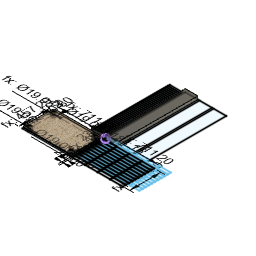
model (Autodesk Fusion 360 design; units mm, degrees)
Autodesk Fusion 360 part; units mm, degrees
sketch "Sketch1" plane through (0, 0, 0) normal (0, 0, 1) x (1, 0, 0) in component "stock"
  line L0 (0, 0) -> (184.15, 0)
  line L1 (184.15, 0) -> (184.15, 1168.4)
  line L2 (184.15, 1168.4) -> (0, 1168.4)
  line L3 (0, 1168.4) -> (0, 0)
  line L4 (-207.15, 0) -> (-23, 0)
  line L5 (-23, 0) -> (-23, 25.4)
  line L6 (-23, 25.4) -> (-207.15, 25.4)
  line L7 (-207.15, 25.4) -> (-207.15, 0)
  line L8 (-207.15, 27.4) -> (-23, 27.4)
  line L9 (-23, 27.4) -> (-23, 52.8)
  line L10 (-207.15, 52.8) -> (-207.15, 27.4)
  line L11 (-23, 52.8) -> (-207.15, 52.8)
  line L12 (-207.15, 54.8) -> (-23, 54.8)
  line L13 (-23, 54.8) -> (-23, 80.2)
  line L14 (-207.15, 80.2) -> (-207.15, 54.8)
  line L15 (-23, 80.2) -> (-207.15, 80.2)
  line L16 (-207.15, 82.2) -> (-23, 82.2)
  line L17 (-23, 82.2) -> (-23, 107.6)
  line L18 (-207.15, 107.6) -> (-207.15, 82.2)
  line L19 (-23, 107.6) -> (-207.15, 107.6)
  line L20 (-207.15, 109.6) -> (-23, 109.6)
  line L21 (-23, 109.6) -> (-23, 135)
  line L22 (-207.15, 135) -> (-207.15, 109.6)
  line L23 (-23, 135) -> (-207.15, 135)
  line L24 (-207.15, 137) -> (-23, 137)
  line L25 (-23, 137) -> (-23, 162.4)
  line L26 (-207.15, 162.4) -> (-207.15, 137)
  line L27 (-23, 162.4) -> (-207.15, 162.4)
  line L28 (-207.15, 164.4) -> (-23, 164.4)
  line L29 (-23, 164.4) -> (-23, 189.8)
  line L30 (-207.15, 189.8) -> (-207.15, 164.4)
  line L31 (-23, 189.8) -> (-207.15, 189.8)
  line L32 (-207.15, 191.8) -> (-23, 191.8)
  line L33 (-23, 191.8) -> (-23, 217.2)
  line L34 (-207.15, 217.2) -> (-207.15, 191.8)
  line L35 (-23, 217.2) -> (-207.15, 217.2)
  line L36 (-207.15, 219.2) -> (-23, 219.2)
  line L37 (-23, 219.2) -> (-23, 244.6)
  line L38 (-207.15, 244.6) -> (-207.15, 219.2)
  line L39 (-23, 244.6) -> (-207.15, 244.6)
  line L40 (-207.15, 246.6) -> (-23, 246.6)
  line L41 (-23, 246.6) -> (-23, 272)
  line L42 (-207.15, 272) -> (-207.15, 246.6)
  line L43 (-23, 272) -> (-207.15, 272)
  line L44 (-207.15, 274) -> (-23, 274)
  line L45 (-23, 274) -> (-23, 299.4)
  line L46 (-207.15, 299.4) -> (-207.15, 274)
  line L47 (-23, 299.4) -> (-207.15, 299.4)
  line L48 (-207.15, 301.4) -> (-23, 301.4)
  line L49 (-23, 301.4) -> (-23, 326.8)
  line L50 (-207.15, 326.8) -> (-207.15, 301.4)
  line L51 (-23, 326.8) -> (-207.15, 326.8)
  line L52 (-207.15, 328.8) -> (-23, 328.8)
  line L53 (-23, 328.8) -> (-23, 354.2)
  line L54 (-207.15, 354.2) -> (-207.15, 328.8)
  line L55 (-23, 354.2) -> (-207.15, 354.2)
  line L56 (-207.15, 356.2) -> (-23, 356.2)
  line L57 (-23, 356.2) -> (-23, 381.6)
  line L58 (-207.15, 381.6) -> (-207.15, 356.2)
  line L59 (-23, 381.6) -> (-207.15, 381.6)
  line L60 (-207.15, 383.6) -> (-23, 383.6)
  line L61 (-23, 383.6) -> (-23, 409)
  line L62 (-207.15, 409) -> (-207.15, 383.6)
  line L63 (-23, 409) -> (-207.15, 409)
  line L64 (-207.15, 411) -> (-23, 411)
  line L65 (-23, 411) -> (-23, 436.4)
  line L66 (-207.15, 436.4) -> (-207.15, 411)
  line L67 (-23, 436.4) -> (-207.15, 436.4)
  line L68 (-207.15, 438.4) -> (-23, 438.4)
  line L69 (-23, 438.4) -> (-23, 463.8)
  line L70 (-207.15, 463.8) -> (-207.15, 438.4)
  line L71 (-23, 463.8) -> (-207.15, 463.8)
  line L72 (-207.15, 465.8) -> (-23, 465.8)
  line L73 (-23, 465.8) -> (-23, 491.2)
  line L74 (-207.15, 491.2) -> (-207.15, 465.8)
  line L75 (-23, 491.2) -> (-207.15, 491.2)
  line L76 (-207.15, 493.2) -> (-23, 493.2)
  line L77 (-23, 493.2) -> (-23, 518.6)
  line L78 (-207.15, 518.6) -> (-207.15, 493.2)
  line L79 (-23, 518.6) -> (-207.15, 518.6)
  line L80 (-207.15, 520.6) -> (-23, 520.6)
  line L81 (-23, 520.6) -> (-23, 546)
  line L82 (-207.15, 546) -> (-207.15, 520.6)
  line L83 (-23, 546) -> (-207.15, 546)
  line L84 (-207.15, 548) -> (-23, 548)
  line L85 (-23, 548) -> (-23, 573.4)
  line L86 (-207.15, 573.4) -> (-207.15, 548)
  line L87 (-23, 573.4) -> (-207.15, 573.4)
  line L88 (-207.15, 575.4) -> (-23, 575.4)
  line L89 (-23, 575.4) -> (-23, 600.8)
  line L90 (-207.15, 600.8) -> (-207.15, 575.4)
  line L91 (-23, 600.8) -> (-207.15, 600.8)
  line L92 (-207.15, 602.8) -> (-23, 602.8)
  line L93 (-23, 602.8) -> (-23, 628.2)
  line L94 (-207.15, 628.2) -> (-207.15, 602.8)
  line L95 (-23, 628.2) -> (-207.15, 628.2)
  line L96 (-207.15, 630.2) -> (-23, 630.2)
  line L97 (-23, 630.2) -> (-23, 655.6)
  line L98 (-207.15, 655.6) -> (-207.15, 630.2)
  line L99 (-23, 655.6) -> (-207.15, 655.6)
  line L100 (-207.15, 657.6) -> (-23, 657.6)
  line L101 (-23, 657.6) -> (-23, 683)
  line L102 (-207.15, 683) -> (-207.15, 657.6)
  line L103 (-23, 683) -> (-207.15, 683)
  line L104 (-207.15, 685) -> (-23, 685)
  line L105 (-23, 685) -> (-23, 710.4)
  line L106 (-207.15, 710.4) -> (-207.15, 685)
  line L107 (-23, 710.4) -> (-207.15, 710.4)
  line L108 (-207.15, 712.4) -> (-23, 712.4)
  line L109 (-23, 712.4) -> (-23, 737.8)
  line L110 (-207.15, 737.8) -> (-207.15, 712.4)
  line L111 (-23, 737.8) -> (-207.15, 737.8)
  line L112 (-207.15, 739.8) -> (-23, 739.8)
  line L113 (-23, 739.8) -> (-23, 765.2)
  line L114 (-207.15, 765.2) -> (-207.15, 739.8)
  line L115 (-23, 765.2) -> (-207.15, 765.2)
  line L116 (-207.15, 767.2) -> (-23, 767.2)
  line L117 (-23, 767.2) -> (-23, 792.6)
  line L118 (-207.15, 792.6) -> (-207.15, 767.2)
  line L119 (-23, 792.6) -> (-207.15, 792.6)
  line L120 (-207.15, 794.6) -> (-23, 794.6)
  line L121 (-23, 794.6) -> (-23, 820)
  line L122 (-207.15, 820) -> (-207.15, 794.6)
  line L123 (-23, 820) -> (-207.15, 820)
  line L124 (-207.15, 822) -> (-23, 822)
  line L125 (-23, 822) -> (-23, 847.4)
  line L126 (-207.15, 847.4) -> (-207.15, 822)
  line L127 (-23, 847.4) -> (-207.15, 847.4)
  line L128 (-207.15, 849.4) -> (-23, 849.4)
  line L129 (-23, 849.4) -> (-23, 874.8)
  line L130 (-207.15, 874.8) -> (-207.15, 849.4)
  line L131 (-23, 874.8) -> (-207.15, 874.8)
  line L132 (-207.15, 876.8) -> (-23, 876.8)
  line L133 (-23, 876.8) -> (-23, 902.2)
  line L134 (-207.15, 902.2) -> (-207.15, 876.8)
  line L135 (-23, 902.2) -> (-207.15, 902.2)
  line L136 (207.15, 1168.4) -> (207.15, 0)
  line L137 (207.15, 0) -> (391.3, 0)
  line L138 (391.3, 1168.4) -> (207.15, 1168.4)
  line L139 (391.3, 0) -> (391.3, 1168.4)
  line L140 (414.3, 1168.4) -> (414.3, 0)
  line L141 (414.3, 0) -> (598.45, 0)
  line L142 (598.45, 1168.4) -> (414.3, 1168.4)
  line L143 (598.45, 0) -> (598.45, 1168.4)
  line L144 (-207.15, 904.2) -> (-23, 904.2)
  line L145 (-23, 904.2) -> (-23, 929.6)
  line L146 (-207.15, 929.6) -> (-207.15, 904.2)
  line L147 (-23, 929.6) -> (-207.15, 929.6)
  line L148 (-207.15, 931.6) -> (-23, 931.6)
  line L149 (-23, 931.6) -> (-23, 957)
  line L150 (-207.15, 957) -> (-207.15, 931.6)
  line L151 (-23, 957) -> (-207.15, 957)
  line L152 (-207.15, 959) -> (-23, 959)
  line L153 (-23, 959) -> (-23, 984.4)
  line L154 (-207.15, 984.4) -> (-207.15, 959)
  line L155 (-23, 984.4) -> (-207.15, 984.4)
  line L156 (-207.15, 986.4) -> (-23, 986.4)
  line L157 (-23, 986.4) -> (-23, 1011.8)
  line L158 (-207.15, 1011.8) -> (-207.15, 986.4)
  line L159 (-23, 1011.8) -> (-207.15, 1011.8)
  line L160 (-207.15, 1013.8) -> (-23, 1013.8)
  line L161 (-23, 1013.8) -> (-23, 1039.2)
  line L162 (-207.15, 1039.2) -> (-207.15, 1013.8)
  line L163 (-23, 1039.2) -> (-207.15, 1039.2)
  line L164 (-207.15, 1041.2) -> (-23, 1041.2)
  line L165 (-23, 1041.2) -> (-23, 1066.6)
  line L166 (-207.15, 1066.6) -> (-207.15, 1041.2)
  line L167 (-23, 1066.6) -> (-207.15, 1066.6)
  line L168 (-207.15, 1068.6) -> (-23, 1068.6)
  line L169 (-23, 1068.6) -> (-23, 1094)
  line L170 (-207.15, 1094) -> (-207.15, 1068.6)
  line L171 (-23, 1094) -> (-207.15, 1094)
  line L172 (-207.15, 1096) -> (-23, 1096)
  line L173 (-23, 1096) -> (-23, 1121.4)
  line L174 (-207.15, 1121.4) -> (-207.15, 1096)
  line L175 (-23, 1121.4) -> (-207.15, 1121.4)
  line L176 (-207.15, 1123.4) -> (-23, 1123.4)
  line L177 (-23, 1123.4) -> (-23, 1148.8)
  line L178 (-207.15, 1148.8) -> (-207.15, 1123.4)
  line L179 (-23, 1148.8) -> (-207.15, 1148.8)
  dimension "d4" = 184.15
  dimension "d5" = 1168.4
  dimension "d19" = 184.15
  dimension "d20" = 25.4
  dimension "d25" = 0
  dimension "d26" = 27.4
  dimension "d27" = 23
  dimension "d30" = 207.15
  dimension "d31" = 0
  constraint horizontal L0
  constraint vertical L1
  constraint horizontal L2
  constraint vertical L3
  constraint coincident L0.start L3.end
  constraint horizontal L4
  constraint vertical L5
  constraint horizontal L6
  constraint vertical L7
  constraint collinear L0 L4
  measures "d4" distance of L1.end L2.end
  measures "d5" distance of L0.start L2.end
  measures "d19" distance of L4.start L4.end
  measures "d20" distance of L4.start L6.end
  measures "d27" distance of L3 L5
sketch "Sketch1 (2)" plane through (0, 0, 0) normal (0, 0, 1) x (1, 0, 0) in component "board"
  line L0 (-734.2, -480.2) -> (-23, -480.2)
  line L1 (-23, -480.2) -> (-23, -23)
  line L2 (-23, -23) -> (-734.2, -23)
  line L3 (-734.2, -23) -> (-734.2, -480.2)
  line L4 (0, -23) -> (184.15, -23)
  line L5 (184.15, -23) -> (184.15, -69.0375)
  line L6 (184.15, -69.0375) -> (0, -69.0375)
  line L7 (0, -69.0375) -> (0, -23)
  line L8 (0, -23) -> (711.2, -23) construction
  line L9 (711.2, -23) -> (711.2, -480.2) construction
  line L10 (711.2, -480.2) -> (0, -480.2) construction
  line L11 (0, -480.2) -> (0, -23) construction
  line L12 (184.15, -69.0375) -> (184.15, -23)
  line L13 (184.15, -23) -> (368.3, -23)
  line L14 (368.3, -69.0375) -> (184.15, -69.0375)
  line L15 (368.3, -23) -> (368.3, -69.0375)
  line L16 (368.3, -69.0375) -> (368.3, -23)
  line L17 (368.3, -23) -> (552.45, -23)
  line L18 (552.45, -69.0375) -> (368.3, -69.0375)
  line L19 (552.45, -23) -> (552.45, -69.0375)
  line L20 (552.45, -69.0375) -> (552.45, -23)
  line L21 (552.45, -23) -> (736.6, -23)
  line L22 (736.6, -69.0375) -> (552.45, -69.0375)
  line L23 (736.6, -23) -> (736.6, -69.0375)
  line L24 (0, -115.075) -> (0, -69.0375)
  line L25 (0, -69.0375) -> (184.15, -69.0375)
  line L26 (184.15, -115.075) -> (0, -115.075)
  line L27 (184.15, -69.0375) -> (184.15, -115.075)
  line L28 (184.15, -115.075) -> (184.15, -69.0375)
  line L29 (184.15, -69.0375) -> (368.3, -69.0375)
  line L30 (368.3, -115.075) -> (184.15, -115.075)
  line L31 (368.3, -69.0375) -> (368.3, -115.075)
  line L32 (368.3, -115.075) -> (368.3, -69.0375)
  line L33 (368.3, -69.0375) -> (552.45, -69.0375)
  line L34 (552.45, -115.075) -> (368.3, -115.075)
  line L35 (552.45, -69.0375) -> (552.45, -115.075)
  line L36 (552.45, -115.075) -> (552.45, -69.0375)
  line L37 (552.45, -69.0375) -> (736.6, -69.0375)
  line L38 (736.6, -115.075) -> (552.45, -115.075)
  line L39 (736.6, -69.0375) -> (736.6, -115.075)
  line L40 (0, -161.1125) -> (0, -115.075)
  line L41 (0, -115.075) -> (184.15, -115.075)
  line L42 (184.15, -161.1125) -> (0, -161.1125)
  line L43 (184.15, -115.075) -> (184.15, -161.1125)
  line L44 (184.15, -161.1125) -> (184.15, -115.075)
  line L45 (184.15, -115.075) -> (368.3, -115.075)
  line L46 (368.3, -161.1125) -> (184.15, -161.1125)
  line L47 (368.3, -115.075) -> (368.3, -161.1125)
  line L48 (368.3, -161.1125) -> (368.3, -115.075)
  line L49 (368.3, -115.075) -> (552.45, -115.075)
  line L50 (552.45, -161.1125) -> (368.3, -161.1125)
  line L51 (552.45, -115.075) -> (552.45, -161.1125)
  line L52 (552.45, -161.1125) -> (552.45, -115.075)
  line L53 (552.45, -115.075) -> (736.6, -115.075)
  line L54 (736.6, -161.1125) -> (552.45, -161.1125)
  line L55 (736.6, -115.075) -> (736.6, -161.1125)
  line L56 (0, -207.15) -> (0, -161.1125)
  line L57 (0, -161.1125) -> (184.15, -161.1125)
  line L58 (184.15, -207.15) -> (0, -207.15)
  line L59 (184.15, -161.1125) -> (184.15, -207.15)
  line L60 (184.15, -207.15) -> (184.15, -161.1125)
  line L61 (184.15, -161.1125) -> (368.3, -161.1125)
  line L62 (368.3, -207.15) -> (184.15, -207.15)
  line L63 (368.3, -161.1125) -> (368.3, -207.15)
  line L64 (368.3, -207.15) -> (368.3, -161.1125)
  line L65 (368.3, -161.1125) -> (552.45, -161.1125)
  line L66 (552.45, -207.15) -> (368.3, -207.15)
  line L67 (552.45, -161.1125) -> (552.45, -207.15)
  line L68 (552.45, -207.15) -> (552.45, -161.1125)
  line L69 (552.45, -161.1125) -> (736.6, -161.1125)
  line L70 (736.6, -207.15) -> (552.45, -207.15)
  line L71 (736.6, -161.1125) -> (736.6, -207.15)
  line L72 (0, -253.1875) -> (0, -207.15)
  line L73 (0, -207.15) -> (184.15, -207.15)
  line L74 (184.15, -253.1875) -> (0, -253.1875)
  line L75 (184.15, -207.15) -> (184.15, -253.1875)
  line L76 (184.15, -253.1875) -> (184.15, -207.15)
  line L77 (184.15, -207.15) -> (368.3, -207.15)
  line L78 (368.3, -253.1875) -> (184.15, -253.1875)
  line L79 (368.3, -207.15) -> (368.3, -253.1875)
  line L80 (368.3, -253.1875) -> (368.3, -207.15)
  line L81 (368.3, -207.15) -> (552.45, -207.15)
  line L82 (552.45, -253.1875) -> (368.3, -253.1875)
  line L83 (552.45, -207.15) -> (552.45, -253.1875)
  line L84 (552.45, -253.1875) -> (552.45, -207.15)
  line L85 (552.45, -207.15) -> (736.6, -207.15)
  line L86 (736.6, -253.1875) -> (552.45, -253.1875)
  line L87 (736.6, -207.15) -> (736.6, -253.1875)
  line L88 (0, -299.225) -> (0, -253.1875)
  line L89 (0, -253.1875) -> (184.15, -253.1875)
  line L90 (184.15, -299.225) -> (0, -299.225)
  line L91 (184.15, -253.1875) -> (184.15, -299.225)
  line L92 (184.15, -299.225) -> (184.15, -253.1875)
  line L93 (184.15, -253.1875) -> (368.3, -253.1875)
  line L94 (368.3, -299.225) -> (184.15, -299.225)
  line L95 (368.3, -253.1875) -> (368.3, -299.225)
  line L96 (368.3, -299.225) -> (368.3, -253.1875)
  line L97 (368.3, -253.1875) -> (552.45, -253.1875)
  line L98 (552.45, -299.225) -> (368.3, -299.225)
  line L99 (552.45, -253.1875) -> (552.45, -299.225)
  line L100 (552.45, -299.225) -> (552.45, -253.1875)
  line L101 (552.45, -253.1875) -> (736.6, -253.1875)
  line L102 (736.6, -299.225) -> (552.45, -299.225)
  line L103 (736.6, -253.1875) -> (736.6, -299.225)
  line L104 (0, -345.2625) -> (0, -299.225)
  line L105 (0, -299.225) -> (184.15, -299.225)
  line L106 (184.15, -345.2625) -> (0, -345.2625)
  line L107 (184.15, -299.225) -> (184.15, -345.2625)
  line L108 (184.15, -345.2625) -> (184.15, -299.225)
  line L109 (184.15, -299.225) -> (368.3, -299.225)
  line L110 (368.3, -345.2625) -> (184.15, -345.2625)
  line L111 (368.3, -299.225) -> (368.3, -345.2625)
  line L112 (368.3, -345.2625) -> (368.3, -299.225)
  line L113 (368.3, -299.225) -> (552.45, -299.225)
  line L114 (552.45, -345.2625) -> (368.3, -345.2625)
  line L115 (552.45, -299.225) -> (552.45, -345.2625)
  line L116 (552.45, -345.2625) -> (552.45, -299.225)
  line L117 (552.45, -299.225) -> (736.6, -299.225)
  line L118 (736.6, -345.2625) -> (552.45, -345.2625)
  line L119 (736.6, -299.225) -> (736.6, -345.2625)
  line L120 (0, -391.3) -> (0, -345.2625)
  line L121 (0, -345.2625) -> (184.15, -345.2625)
  line L122 (184.15, -391.3) -> (0, -391.3)
  line L123 (184.15, -345.2625) -> (184.15, -391.3)
  line L124 (184.15, -391.3) -> (184.15, -345.2625)
  line L125 (184.15, -345.2625) -> (368.3, -345.2625)
  line L126 (368.3, -391.3) -> (184.15, -391.3)
  line L127 (368.3, -345.2625) -> (368.3, -391.3)
  line L128 (368.3, -391.3) -> (368.3, -345.2625)
  line L129 (368.3, -345.2625) -> (552.45, -345.2625)
  line L130 (552.45, -391.3) -> (368.3, -391.3)
  line L131 (552.45, -345.2625) -> (552.45, -391.3)
  line L132 (552.45, -391.3) -> (552.45, -345.2625)
  line L133 (552.45, -345.2625) -> (736.6, -345.2625)
  line L134 (736.6, -391.3) -> (552.45, -391.3)
  line L135 (736.6, -345.2625) -> (736.6, -391.3)
  line L136 (0, -437.3375) -> (0, -391.3)
  line L137 (0, -391.3) -> (184.15, -391.3)
  line L138 (184.15, -437.3375) -> (0, -437.3375)
  line L139 (184.15, -391.3) -> (184.15, -437.3375)
  line L140 (184.15, -437.3375) -> (184.15, -391.3)
  line L141 (184.15, -391.3) -> (368.3, -391.3)
  line L142 (368.3, -437.3375) -> (184.15, -437.3375)
  line L143 (368.3, -391.3) -> (368.3, -437.3375)
  line L144 (368.3, -437.3375) -> (368.3, -391.3)
  line L145 (368.3, -391.3) -> (552.45, -391.3)
  line L146 (552.45, -437.3375) -> (368.3, -437.3375)
  line L147 (552.45, -391.3) -> (552.45, -437.3375)
  line L148 (552.45, -437.3375) -> (552.45, -391.3)
  line L149 (552.45, -391.3) -> (736.6, -391.3)
  line L150 (736.6, -437.3375) -> (552.45, -437.3375)
  line L151 (736.6, -391.3) -> (736.6, -437.3375)
  line L152 (0, -483.375) -> (0, -437.3375)
  line L153 (0, -437.3375) -> (184.15, -437.3375)
  line L154 (184.15, -483.375) -> (0, -483.375)
  line L155 (184.15, -437.3375) -> (184.15, -483.375)
  line L156 (184.15, -483.375) -> (184.15, -437.3375)
  line L157 (184.15, -437.3375) -> (368.3, -437.3375)
  line L158 (368.3, -483.375) -> (184.15, -483.375)
  line L159 (368.3, -437.3375) -> (368.3, -483.375)
  line L160 (368.3, -483.375) -> (368.3, -437.3375)
  line L161 (368.3, -437.3375) -> (552.45, -437.3375)
  line L162 (552.45, -483.375) -> (368.3, -483.375)
  line L163 (552.45, -437.3375) -> (552.45, -483.375)
  line L164 (552.45, -483.375) -> (552.45, -437.3375)
  line L165 (552.45, -437.3375) -> (736.6, -437.3375)
  line L166 (736.6, -483.375) -> (552.45, -483.375)
  line L167 (736.6, -437.3375) -> (736.6, -483.375)
  line L168 (-683.4, -429.4) -> (-73.8, -429.4) construction
  line L169 (-73.8, -429.4) -> (-73.8, -73.8) construction
  line L170 (-73.8, -73.8) -> (-683.4, -73.8) construction
  line L171 (-683.4, -73.8) -> (-683.4, -429.4) construction
  circle A0 centre (-683.4, -73.8) radius 9.525
  circle A1 centre (-73.8, -73.8) radius 9.525
  circle A2 centre (-73.8, -429.4) radius 9.525
  circle A3 centre (-683.4, -429.4) radius 9.525
  dimension "d14" = 711.2
  dimension "d15" = 457.2
  dimension "d36" = 23
  dimension "d38" = 23
  dimension "d39" = 184.15
  dimension "d40" = 46.0375
  dimension "d41" = 23
  dimension "d42" = 711.2
  dimension "d43" = 457.2
  dimension "d46" = 184.15
  dimension "d79" = 19.05
  dimension "d80" = 19.05
  dimension "d81" = 19.05
  dimension "d82" = 19.05
  constraint horizontal L0
  constraint vertical L1
  constraint horizontal L2
  constraint vertical L3
  constraint horizontal L4
  constraint vertical L5
  constraint horizontal L6
  constraint vertical L7
  constraint collinear L2 L4
  constraint horizontal L8
  constraint vertical L9
  constraint horizontal L10
  constraint vertical L11
  constraint coincident L170.end L171.start
  constraint coincident L169.end L170.start
  constraint coincident L168.end L169.start
  constraint coincident L168.start L171.end
  measures "d14" distance of L1.end L2.end
  measures "d15" distance of L0.start L2.end
  measures "d36" distance of L2 origin
  measures "d38" distance of origin L1
  measures "d39" distance of L4.start L4.end
  measures "d40" distance of L4.start L6.end
  measures "d41" distance of L1 L7
  measures "d42" distance of L4.start L8.end
  measures "d43" distance of L8.end L9.end
  measures "d79" diameter of A0
  measures "d80" diameter of A1
  measures "d81" diameter of A3
  measures "d82" diameter of A2
extrude "Extrude2" add sketch "Sketch1" along normal blind 46.0375 contours L0 L1 L2 L3 makes body 1 in component "stock"
extrude "Extrude3" add sketch "Sketch1" along normal blind 46.0375 separate body contours L4 L5 L6 L7 makes body 2 in component "stock"
sketch "Sketch2" plane through (0, 0, 0) normal (0, 0, 1) x (1, 0, 0) in component "actual"
  line L0 (0, 0) -> (129.54, 0)
  line L1 (129.54, 0) -> (129.54, 46.0375)
  line L2 (129.54, 46.0375) -> (0, 46.0375)
  line L3 (0, 46.0375) -> (0, 0)
  line L4 (129.54, 0) -> (302.26, 0)
  line L5 (302.26, 0) -> (302.26, 46.0375)
  line L6 (302.26, 46.0375) -> (129.54, 46.0375)
  line L7 (129.54, 46.0375) -> (129.54, 0)
  line L8 (302.26, 0) -> (431.8, 0)
  line L9 (431.8, 0) -> (431.8, 46.0375)
  line L10 (431.8, 46.0375) -> (302.26, 46.0375)
  line L11 (302.26, 46.0375) -> (302.26, 0)
  line L12 (431.8, 0) -> (584.2, 0)
  line L13 (584.2, 0) -> (584.2, 46.0375)
  line L14 (584.2, 46.0375) -> (431.8, 46.0375)
  line L15 (431.8, 46.0375) -> (431.8, 0)
  line L16 (584.2, 0) -> (736.6, 0)
  line L17 (736.6, 0) -> (736.6, 46.0375)
  line L18 (736.6, 46.0375) -> (584.2, 46.0375)
  line L19 (584.2, 46.0375) -> (584.2, 0)
  line L20 (736.6, 0) -> (909.32, 0)
  line L21 (909.32, 0) -> (909.32, 46.0375)
  line L22 (909.32, 46.0375) -> (736.6, 46.0375)
  line L23 (736.6, 46.0375) -> (736.6, 0)
  line L24 (606.82, -46.0375) -> (779.54, -46.0375)
  line L25 (324.88, 0) -> (172.48, 0)
  line L26 (606.82, -46.0375) -> (606.82, 0)
  line L27 (477.28, 0) -> (477.28, -46.0375)
  line L28 (324.88, 0) -> (324.88, -46.0375)
  line L29 (324.88, -46.0375) -> (477.28, -46.0375)
  line L30 (172.48, 0) -> (-0.24, 0)
  line L31 (477.28, 0) -> (324.88, 0)
  line L32 (-0.24, 0) -> (-0.24, -46.0375)
  line L33 (-0.24, -46.0375) -> (172.48, -46.0375)
  line L34 (172.48, -46.0375) -> (172.48, 0)
  line L35 (172.48, 0) -> (172.48, -46.0375)
  line L36 (324.88, -46.0375) -> (324.88, 0)
  line L37 (779.54, -46.0375) -> (909.08, -46.0375)
  line L38 (779.54, -46.0375) -> (779.54, 0)
  line L39 (477.28, -46.0375) -> (606.82, -46.0375)
  line L40 (909.08, 0) -> (779.54, 0)
  line L41 (909.08, -46.0375) -> (909.08, 0)
  line L42 (606.82, 0) -> (477.28, 0)
  line L43 (779.54, 0) -> (606.82, 0)
  line L44 (779.54, 0) -> (779.54, -46.0375)
  line L45 (606.82, 0) -> (606.82, -46.0375)
  line L46 (172.48, -46.0375) -> (324.88, -46.0375)
  line L47 (477.28, -46.0375) -> (477.28, 0)
  line L48 (-0.24, -138.1125) -> (172.48, -138.1125)
  line L49 (324.88, -92.075) -> (324.88, -138.1125)
  line L50 (129.54, -46.0375) -> (0, -46.0375)
  line L51 (584.2, -92.075) -> (736.6, -92.075)
  line L52 (431.8, -92.075) -> (584.2, -92.075)
  line L53 (324.88, -92.075) -> (172.48, -92.075)
  line L54 (477.28, -138.1125) -> (606.82, -138.1125)
  line L55 (584.2, -46.0375) -> (584.2, -92.075)
  line L56 (606.82, -92.075) -> (477.28, -92.075)
  line L57 (584.2, -92.075) -> (584.2, -46.0375)
  line L58 (324.88, -138.1125) -> (324.88, -92.075)
  line L59 (172.48, -92.075) -> (172.48, -138.1125)
  line L60 (302.26, -92.075) -> (302.26, -46.0375)
  line L61 (736.6, -46.0375) -> (584.2, -46.0375)
  line L62 (736.6, -92.075) -> (909.32, -92.075)
  line L63 (606.82, -92.075) -> (606.82, -138.1125)
  line L64 (736.6, -92.075) -> (736.6, -46.0375)
  line L65 (909.32, -92.075) -> (909.32, -46.0375)
  line L66 (909.08, -138.1125) -> (909.08, -92.075)
  line L67 (909.32, -46.0375) -> (736.6, -46.0375)
  line L68 (736.6, -46.0375) -> (736.6, -92.075)
  line L69 (606.82, -138.1125) -> (606.82, -92.075)
  line L70 (779.54, -138.1125) -> (909.08, -138.1125)
  line L71 (779.54, -92.075) -> (606.82, -92.075)
  line L72 (779.54, -138.1125) -> (779.54, -92.075)
  line L73 (909.08, -92.075) -> (779.54, -92.075)
  line L74 (779.54, -92.075) -> (779.54, -138.1125)
  line L75 (606.82, -138.1125) -> (779.54, -138.1125)
  line L76 (172.48, -138.1125) -> (324.88, -138.1125)
  line L77 (129.54, -92.075) -> (302.26, -92.075)
  line L78 (477.28, -138.1125) -> (477.28, -92.075)
  line L79 (302.26, -46.0375) -> (129.54, -46.0375)
  line L80 (172.48, -92.075) -> (-0.24, -92.075)
  line L81 (431.8, -92.075) -> (431.8, -46.0375)
  line L82 (477.28, -92.075) -> (324.88, -92.075)
  line L83 (431.8, -46.0375) -> (302.26, -46.0375)
  line L84 (477.28, -92.075) -> (477.28, -138.1125)
  line L85 (129.54, -92.075) -> (129.54, -46.0375)
  line L86 (0, -92.075) -> (129.54, -92.075)
  line L87 (0, -46.0375) -> (0, -92.075)
  line L88 (302.26, -46.0375) -> (302.26, -92.075)
  line L89 (584.2, -46.0375) -> (431.8, -46.0375)
  line L90 (172.48, -138.1125) -> (172.48, -92.075)
  line L91 (129.54, -46.0375) -> (129.54, -92.075)
  line L92 (431.8, -46.0375) -> (431.8, -92.075)
  line L93 (-0.24, -92.075) -> (-0.24, -138.1125)
  line L94 (302.26, -92.075) -> (431.8, -92.075)
  line L95 (324.88, -138.1125) -> (477.28, -138.1125)
  line L96 (-0.24, -230.1875) -> (172.48, -230.1875)
  line L97 (324.88, -184.15) -> (324.88, -230.1875)
  line L98 (129.54, -138.1125) -> (0, -138.1125)
  line L99 (584.2, -184.15) -> (736.6, -184.15)
  line L100 (431.8, -184.15) -> (584.2, -184.15)
  line L101 (324.88, -184.15) -> (172.48, -184.15)
  line L102 (477.28, -230.1875) -> (606.82, -230.1875)
  line L103 (584.2, -138.1125) -> (584.2, -184.15)
  line L104 (606.82, -184.15) -> (477.28, -184.15)
  line L105 (584.2, -184.15) -> (584.2, -138.1125)
  line L106 (324.88, -230.1875) -> (324.88, -184.15)
  line L107 (172.48, -184.15) -> (172.48, -230.1875)
  line L108 (302.26, -184.15) -> (302.26, -138.1125)
  line L109 (736.6, -138.1125) -> (584.2, -138.1125)
  line L110 (736.6, -184.15) -> (909.32, -184.15)
  line L111 (606.82, -184.15) -> (606.82, -230.1875)
  line L112 (736.6, -184.15) -> (736.6, -138.1125)
  line L113 (909.32, -184.15) -> (909.32, -138.1125)
  line L114 (909.08, -230.1875) -> (909.08, -184.15)
  line L115 (909.32, -138.1125) -> (736.6, -138.1125)
  line L116 (736.6, -138.1125) -> (736.6, -184.15)
  line L117 (606.82, -230.1875) -> (606.82, -184.15)
  line L118 (779.54, -230.1875) -> (909.08, -230.1875)
  line L119 (779.54, -184.15) -> (606.82, -184.15)
  line L120 (779.54, -230.1875) -> (779.54, -184.15)
  line L121 (909.08, -184.15) -> (779.54, -184.15)
  line L122 (779.54, -184.15) -> (779.54, -230.1875)
  line L123 (606.82, -230.1875) -> (779.54, -230.1875)
  line L124 (172.48, -230.1875) -> (324.88, -230.1875)
  line L125 (129.54, -184.15) -> (302.26, -184.15)
  line L126 (477.28, -230.1875) -> (477.28, -184.15)
  line L127 (302.26, -138.1125) -> (129.54, -138.1125)
  line L128 (172.48, -184.15) -> (-0.24, -184.15)
  line L129 (431.8, -184.15) -> (431.8, -138.1125)
  line L130 (477.28, -184.15) -> (324.88, -184.15)
  line L131 (431.8, -138.1125) -> (302.26, -138.1125)
  line L132 (477.28, -184.15) -> (477.28, -230.1875)
  line L133 (129.54, -184.15) -> (129.54, -138.1125)
  line L134 (0, -184.15) -> (129.54, -184.15)
  line L135 (0, -138.1125) -> (0, -184.15)
  line L136 (302.26, -138.1125) -> (302.26, -184.15)
  line L137 (584.2, -138.1125) -> (431.8, -138.1125)
  line L138 (172.48, -230.1875) -> (172.48, -184.15)
  line L139 (129.54, -138.1125) -> (129.54, -184.15)
  line L140 (431.8, -138.1125) -> (431.8, -184.15)
  line L141 (-0.24, -184.15) -> (-0.24, -230.1875)
  line L142 (302.26, -184.15) -> (431.8, -184.15)
  line L143 (324.88, -230.1875) -> (477.28, -230.1875)
  line L144 (-0.24, -322.2625) -> (172.48, -322.2625)
  line L145 (324.88, -276.225) -> (324.88, -322.2625)
  line L146 (129.54, -230.1875) -> (0, -230.1875)
  line L147 (584.2, -276.225) -> (736.6, -276.225)
  line L148 (431.8, -276.225) -> (584.2, -276.225)
  line L149 (324.88, -276.225) -> (172.48, -276.225)
  line L150 (477.28, -322.2625) -> (606.82, -322.2625)
  line L151 (584.2, -230.1875) -> (584.2, -276.225)
  line L152 (606.82, -276.225) -> (477.28, -276.225)
  line L153 (584.2, -276.225) -> (584.2, -230.1875)
  line L154 (324.88, -322.2625) -> (324.88, -276.225)
  line L155 (172.48, -276.225) -> (172.48, -322.2625)
  line L156 (302.26, -276.225) -> (302.26, -230.1875)
  line L157 (736.6, -230.1875) -> (584.2, -230.1875)
  line L158 (736.6, -276.225) -> (909.32, -276.225)
  line L159 (606.82, -276.225) -> (606.82, -322.2625)
  line L160 (736.6, -276.225) -> (736.6, -230.1875)
  line L161 (909.32, -276.225) -> (909.32, -230.1875)
  line L162 (909.08, -322.2625) -> (909.08, -276.225)
  line L163 (909.32, -230.1875) -> (736.6, -230.1875)
  line L164 (736.6, -230.1875) -> (736.6, -276.225)
  line L165 (606.82, -322.2625) -> (606.82, -276.225)
  line L166 (779.54, -322.2625) -> (909.08, -322.2625)
  line L167 (779.54, -276.225) -> (606.82, -276.225)
  line L168 (779.54, -322.2625) -> (779.54, -276.225)
  line L169 (909.08, -276.225) -> (779.54, -276.225)
  line L170 (779.54, -276.225) -> (779.54, -322.2625)
  line L171 (606.82, -322.2625) -> (779.54, -322.2625)
  line L172 (172.48, -322.2625) -> (324.88, -322.2625)
  line L173 (129.54, -276.225) -> (302.26, -276.225)
  line L174 (477.28, -322.2625) -> (477.28, -276.225)
  line L175 (302.26, -230.1875) -> (129.54, -230.1875)
  line L176 (172.48, -276.225) -> (-0.24, -276.225)
  line L177 (431.8, -276.225) -> (431.8, -230.1875)
  line L178 (477.28, -276.225) -> (324.88, -276.225)
  line L179 (431.8, -230.1875) -> (302.26, -230.1875)
  line L180 (477.28, -276.225) -> (477.28, -322.2625)
  line L181 (129.54, -276.225) -> (129.54, -230.1875)
  line L182 (0, -276.225) -> (129.54, -276.225)
  line L183 (0, -230.1875) -> (0, -276.225)
  line L184 (302.26, -230.1875) -> (302.26, -276.225)
  line L185 (584.2, -230.1875) -> (431.8, -230.1875)
  line L186 (172.48, -322.2625) -> (172.48, -276.225)
  line L187 (129.54, -230.1875) -> (129.54, -276.225)
  line L188 (431.8, -230.1875) -> (431.8, -276.225)
  line L189 (-0.24, -276.225) -> (-0.24, -322.2625)
  line L190 (302.26, -276.225) -> (431.8, -276.225)
  line L191 (324.88, -322.2625) -> (477.28, -322.2625)
  line L192 (-0.24, -414.3375) -> (172.48, -414.3375)
  line L193 (324.88, -368.3) -> (324.88, -414.3375)
  line L194 (129.54, -322.2625) -> (0, -322.2625)
  line L195 (584.2, -368.3) -> (736.6, -368.3)
  line L196 (431.8, -368.3) -> (584.2, -368.3)
  line L197 (324.88, -368.3) -> (172.48, -368.3)
  line L198 (477.28, -414.3375) -> (606.82, -414.3375)
  line L199 (584.2, -322.2625) -> (584.2, -368.3)
  line L200 (606.82, -368.3) -> (477.28, -368.3)
  line L201 (584.2, -368.3) -> (584.2, -322.2625)
  line L202 (324.88, -414.3375) -> (324.88, -368.3)
  line L203 (172.48, -368.3) -> (172.48, -414.3375)
  line L204 (302.26, -368.3) -> (302.26, -322.2625)
  line L205 (736.6, -322.2625) -> (584.2, -322.2625)
  line L206 (736.6, -368.3) -> (909.32, -368.3)
  line L207 (606.82, -368.3) -> (606.82, -414.3375)
  line L208 (736.6, -368.3) -> (736.6, -322.2625)
  line L209 (909.32, -368.3) -> (909.32, -322.2625)
  line L210 (909.08, -414.3375) -> (909.08, -368.3)
  line L211 (909.32, -322.2625) -> (736.6, -322.2625)
  line L212 (736.6, -322.2625) -> (736.6, -368.3)
  line L213 (606.82, -414.3375) -> (606.82, -368.3)
  line L214 (779.54, -414.3375) -> (909.08, -414.3375)
  line L215 (779.54, -368.3) -> (606.82, -368.3)
  line L216 (779.54, -414.3375) -> (779.54, -368.3)
  line L217 (909.08, -368.3) -> (779.54, -368.3)
  line L218 (779.54, -368.3) -> (779.54, -414.3375)
  line L219 (606.82, -414.3375) -> (779.54, -414.3375)
  line L220 (172.48, -414.3375) -> (324.88, -414.3375)
  line L221 (129.54, -368.3) -> (302.26, -368.3)
  line L222 (477.28, -414.3375) -> (477.28, -368.3)
  line L223 (302.26, -322.2625) -> (129.54, -322.2625)
  line L224 (172.48, -368.3) -> (-0.24, -368.3)
  line L225 (431.8, -368.3) -> (431.8, -322.2625)
  line L226 (477.28, -368.3) -> (324.88, -368.3)
  line L227 (431.8, -322.2625) -> (302.26, -322.2625)
  line L228 (477.28, -368.3) -> (477.28, -414.3375)
  line L229 (129.54, -368.3) -> (129.54, -322.2625)
  line L230 (0, -368.3) -> (129.54, -368.3)
  line L231 (0, -322.2625) -> (0, -368.3)
  line L232 (302.26, -322.2625) -> (302.26, -368.3)
  line L233 (584.2, -322.2625) -> (431.8, -322.2625)
  line L234 (172.48, -414.3375) -> (172.48, -368.3)
  line L235 (129.54, -322.2625) -> (129.54, -368.3)
  line L236 (431.8, -322.2625) -> (431.8, -368.3)
  line L237 (-0.24, -368.3) -> (-0.24, -414.3375)
  line L238 (302.26, -368.3) -> (431.8, -368.3)
  line L239 (324.88, -414.3375) -> (477.28, -414.3375)
  point P0 (0, -92.075)
  point P1 (0, -184.15)
  point P2 (0, -276.225)
  point P3 (0, -368.3)
  dimension "d56" = 46.0375
  dimension "d57" = 129.54
  dimension "d58" = 172.72
  dimension "d59" = 129.54
  dimension "d60" = 152.4
  dimension "d61" = 152.4
  dimension "d62" = 172.72
  dimension "d63" = 46.0375
  dimension "d64" = 129.54
  dimension "d65" = 172.72
  dimension "d66" = 129.54
  dimension "d67" = 152.4
  dimension "d68" = 152.4
  dimension "d69" = 172.72
  dimension "d72" = 0
  dimension "d73" = -368.3
  constraint horizontal L0
  constraint vertical L1
  constraint horizontal L2
  constraint vertical L3
  constraint horizontal L4
  constraint vertical L5
  constraint horizontal L6
  constraint vertical L7
  constraint horizontal L8
  constraint vertical L9
  constraint horizontal L10
  constraint vertical L11
  constraint horizontal L12
  constraint vertical L13
  constraint horizontal L14
  constraint vertical L15
  constraint horizontal L16
  constraint vertical L17
  constraint horizontal L18
  constraint vertical L19
  constraint horizontal L20
  constraint vertical L21
  constraint horizontal L22
  constraint vertical L23
  constraint collinear L2 L6
  constraint collinear L6 L10
  constraint collinear L10 L14
  constraint collinear L14 L18
  constraint collinear L18 L22
  constraint collinear L24 L37
  constraint collinear L24 L39
  constraint collinear L29 L39
  constraint collinear L29 L46
  constraint collinear L33 L46
  measures "d56" distance of L0.start L2.end
  measures "d57" distance of L1.end L2.end
  measures "d58" distance of L5.end L1.end
  measures "d59" distance of L9.end L5.end
  measures "d60" distance of L13.end L9.end
  measures "d61" distance of L17.end L13.end
  measures "d62" distance of L21.end L17.end
  measures "d63" distance of L37.end L40.start
  measures "d64" distance of L24.end L37.end
  measures "d65" distance of L24.end L24.start
  measures "d66" distance of L27.end L24.start
  measures "d67" distance of L28.end L27.end
  measures "d68" distance of L33.end L28.end
  measures "d69" distance of L33.end L32.end
extrude "Extrude1" add sketch "Sketch1 (2)" along normal blind 25.4 separate body contours L0 L1 L2 L3 | A0 | A1 | A2 | A3 makes body 3
extrude "Extrude2'" add sketch "Sketch1 (2)" against normal blind 5 draft -20 separate body contours A0 | A1 | A2 | A3 makes body 4 at (-79.3605, -422.4273, -1.6667) makes body 5 at (-69.3408, -81.5235, -1.6667) makes body 6 at (-684.0665, -420.5066, -1.6667) makes body 7 at (-684.0665, -64.9066, -1.6667)
fillet "Fillet1" radius 3 4 faces at (-73.7146, -434.0337, -5) (-76.2145, -76.1946, -5) (-685.2828, -431.1469, -5) (-678.2649, -75.5583, -5) on bodies 4 5 6 7
fillet "Fillet2" radius 30 4 edges at (-734.2, -480.2, 12.7) (-23, -480.2, 12.7) (-734.2, -23, 12.7) (-23, -23, 12.7) on bodies 3
chamfer "Chamfer1" distance 12 angle 45 8 edges at (-378.6, -480.2, 0) (-31.7868, -471.4132, 0) (-23, -251.6, 0) (-31.7868, -31.7868, 0) (-378.6, -23, 0) (-725.4132, -31.7868, 0) (-734.2, -251.6, 0) (-725.4132, -471.4132, 0) on bodies 3
chamfer "Chamfer2" distance 2 angle 45 8 edges at (-378.6, -480.2, 25.4) (-31.7868, -471.4132, 25.4) (-23, -251.6, 25.4) (-31.7868, -31.7868, 25.4) (-378.6, -23, 25.4) (-725.4132, -31.7868, 25.4) (-734.2, -251.6, 25.4) (-725.4132, -471.4132, 25.4) on bodies 3
component "stock" placed x (1, 0, 0) y (0, 1, 0) z (0, 0, 1) at (0, 0, 0)
component "board" placed x (1, 0, 0) y (0, 1, 0) z (0, 0, 1) at (0, 0, 0)
component "actual" placed x (1, 0, 0) y (0, 1, 0) z (0, 0, 1) at (0, 0, 0)
equation "stockThickness = 1 13/16\""
equation "stockWidth = 7 1/4\""
equation "stockLength = 46\""
equation "d4 = stockWidth"
equation "d5 = stockLength"
equation "boardWidth = 28\""
equation "boardDepth = 18\""
equation "d14 = boardWidth"
equation "d15 = boardDepth"
equation "boardThickness = 1\""
equation "d19 = d4"
equation "d20 = boardThickness"
equation "kerf = 2 mm"
equation "d26 = boardThickness + kerf"
equation "d30 = stockWidth + 23 mm"
equation "d32 = stockThickness"
equation "d34 = stockThickness"
equation "d39 = stockWidth"
equation "d40 = stockThickness"
equation "d41 = d38"
equation "d42 = d14"
equation "d43 = d15"
equation "d46 = stockWidth"
equation "d47 = -stockThickness"
equation "d56 = stockThickness"
equation "d59 = d57"
equation "d60 = 6\""
equation "d61 = d60"
equation "d62 = d58"
equation "d63 = stockThickness"
equation "d66 = d57"
equation "d67 = 6\""
equation "d68 = d60"
equation "d69 = d58"
equation "d73 = -4 * 2 * stockThickness"
equation "d74 = boardThickness"
equation "footInset = 2\""
equation "footDiameter = 3/4\""
equation "d78 = -footInset"
equation "d79 = footDiameter"
equation "d80 = d79"
equation "d81 = d79"
equation "d82 = d79"
